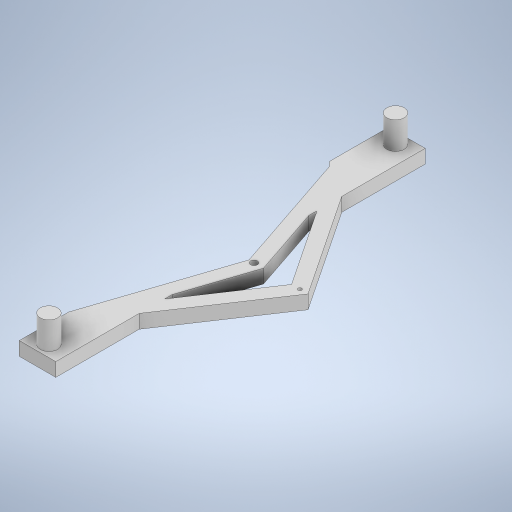
# Autodesk Inventor part: SteeringBaru
Saved by Autodesk Inventor 2024 (Build 280153000, 153)
## iProperties
Created: 2025-12-15
Part Number: SteeringBaru
Material: Generic
Document SubType Name: Modeling
Designer: risda
Density: 1 g/cm^3
Appearance: Default
Author: risda
Autodesk Inventor part; units mm, degrees
ref_plane "YZ Plane" through (0, 0, 0) normal (1, 0, 0) x (0, 1, 0)
ref_plane "XZ Plane" through (0, 0, 0) normal (0, 1, 0) x (-1, 0, 0)
ref_plane "XY Plane" through (0, 0, 0) normal (0, 0, 1) x (1, 0, 0)
sketch "Sketch1" plane through (0, 0, 0) normal (0, 1, 0) x (-1, 0, 0)
  line L0 (0, 0) -> (0, -81)
  line L1 (0, -81) -> (-8, -81)
  line L2 (-8, -81) -> (-8, 0)
  line L3 (0, 0) -> (-8, 0)
  line L4 (-4, 0) -> (-4, -2.5)
  line L5 (-4, -81) -> (-4, -78.5)
  circle A0 centre (-4, -2.5) radius 1.9
  circle A1 centre (-4, -78.5) radius 1.9
  dimension "d0" = 81
  dimension "d1" = 8
  dimension "d2" = 81
  dimension "d3" = 2.5
  dimension "d4" = 2.5
  dimension "d5" = 3.8
  dimension "d6" = 3.8
  constraints: 12 end point, 3 vertical, 2 centre point, 2 coincident, 2 midpoint, 1 horizontal, 1 perpendicular
  measures "d0" distance of L0.start L0.end
  measures "d1" distance of L0.end L1.end
  measures "d2" distance of L1.end L2.end
  measures "d3" distance of L4.start L4.end
  measures "d4" distance of L5.start L5.end
  measures "d5" diameter of A0
  measures "d6" diameter of A1
extrude "Extrusion1" add sketch "Sketch1" along normal blind 3
extrude "Extrusion2" add sketch "Sketch1" along normal blind 9 contours A0 | A1
sketch "Sketch2" plane through (0, 3, 0) normal (0, 1, 0) x (1, 0, 0)
  line L0 (8, 0) -> (8, 81) projected
  line L1 (8, 40.5) -> (18, 40.5)
  line L2 (8, 40.5) -> (8, 25.5)
  line L3 (8, 25.5) -> (0, 25.5)
  line L4 (0, 81) -> (0, 0) projected
  line L5 (8, 40.5) -> (8, 55.5)
  line L6 (8, 55.5) -> (0, 55.5)
  line L7 (0, 55.5) -> (0, 25.5)
  line L8 (8, 25.5) -> (18, 40.5)
  line L9 (8, 55.5) -> (18, 40.5)
  line L10 (8.8321, 24.9453) -> (18.8321, 39.9453)
  line L11 (8.8321, 56.0547) -> (18.8321, 41.0547)
  line L12 (8.8321, 24.9453) -> (8, 23.6972)
  line L13 (8, 23.6972) -> (8, 25.5)
  line L14 (8, 55.5) -> (8, 57.3028)
  line L15 (8.8321, 56.0547) -> (8, 57.3028)
  line L16 (18.8321, 39.9453) -> (19.2019, 40.5)
  line L17 (18.8321, 41.0547) -> (19.2019, 40.5)
  line L18 (5, 25.5) -> (5, 13.7889)
  line L19 (5, 13.7889) -> (11.3282, 23.2812)
  line L20 (11.3282, 23.2812) -> (21.3282, 38.2812)
  line L21 (21.3282, 38.2812) -> (22.8074, 40.5)
  line L22 (22.8074, 40.5) -> (21.3282, 42.7188)
  line L23 (21.3282, 42.7188) -> (11.3282, 57.7188)
  line L24 (11.3282, 57.7188) -> (5, 67.2111)
  line L25 (5, 67.2111) -> (5, 55.5)
  line L26 (8, 23.6972) -> (0, 23.6972)
  line L27 (0, 25.5) -> (0, 23.6972)
  line L28 (8, 57.3028) -> (0, 57.3028)
  line L29 (0, 57.3028) -> (0, 55.5)
  point P0 (8, 18.2889)
  point P1 (8, 62.7111)
  dimension "d11" = 10
  dimension "d12" = 15
  dimension "d13" = 15
  dimension "d14" = 1
  dimension "d15" = 1
  dimension "d16" = 3
  constraints: 56 end point, 9 point on line, 4 collinear, 4 perpendicular, 2 horizontal, 2 parallel, 1 midpoint, 1 vertical, 7 other
  measures "d11" distance of L1.start L1.end
  measures "d12" distance of L1.start L2.end
  measures "d13" distance of L1.start L5.end
  measures "d14" distance between parallel lines of L8 L10
  measures "d15" distance between parallel lines of L9 L11
  measures "d16" distance between parallel lines of L11 L23
extrude "Extrusion3" add sketch "Sketch2" against normal blind 3 contours L12 L10 L16 L17 L11 L15 L0 L24 L23 L22 L21 L20 L19
extrude "Extrusion4" cut sketch "Sketch2" against normal blind 3 contours L26 L18 L3 L0 | L3 L4 L6 L0 | L26 L4 L3 L18 | L6 L25 L28 L0 | L6 L4 L28 L25
chamfer "Chamfer1" distance 3 angle 45 2 edges at (0, 1.5, -57.3028) (0, 1.5, -23.6972)
fillet "Fillet1" radius 1 2 edges at (8, 1.5, -57.3028) (8, 1.5, -23.6972)
sketch "Sketch3" plane through (0, 3, 0) normal (0, 1, 0) x (1, 0, 0)
  line L0 (22.8074, 40.5) -> (8, 62.7111) projected
  line L1 (22.8074, 40.5) -> (21.0044, 40.5)
  circle A0 centre (21.0044, 40.5) radius 0.4
  point P0 (0, 0)
  dimension "d25" = 1.803
  dimension "d26" = 0.8
  constraints: 2 end point, 1 centre point, 1 coincident, 1 horizontal
  measures "d25" distance of L0.start L1.end
  measures "d26" diameter of A0
extrude "Extrusion5" cut sketch "Sketch3" against normal blind 3
sketch "Sketch4" plane through (0, 3, 0) normal (0, 1, 0) x (1, 0, 0)
  line L0 (0, 57.3028) -> (8.0349, 57.3028)
  line L1 (0, 57.3028) -> (0, 23.6972)
  line L2 (0, 23.6972) -> (8.0349, 23.6972)
  line L3 (8.0349, 23.6972) -> (8.0349, 57.3028)
  line L4 (0, 60.3028) -> (3, 57.3028) projected
  line L5 (0, 57.3028) -> (0, 60.3028)
  line L6 (0, 60.3028) -> (3, 57.3028)
  line L7 (0, 20.6972) -> (0, 0) projected
  line L8 (0, 20.6972) -> (0, 23.6972)
  line L9 (0, 20.6972) -> (3, 23.6972)
  line L10 (0, 57.3028) -> (8, 57.3028)
  line L11 (8, 57.3028) -> (8, 55.5125)
  line L12 (8, 55.5125) -> (0, 55.5125)
  line L13 (0, 55.5125) -> (0, 57.3028)
  line L14 (8, 55.5125) -> (13.0424, 40.5013)
  line L15 (13.0424, 40.5013) -> (8.0349, 25.4511)
  line L16 (4.5889, 24.5965) -> (9.8792, 40.4967)
  line L17 (9.8792, 40.4967) -> (4.5467, 56.3715)
  circle A0 centre (10.9842, 40.4967) radius 0.75
  line L18 (9.8792, 40.4967) -> (8.0349, 40.5)
  line L19 (9.8792, 40.4967) -> (10.9842, 40.4967)
  point P0 (8.0349, 45.9872)
  point P1 (8.0349, 34.9536)
  dimension "d29" = 8
  dimension "d30" = 3
  dimension "d31" = 1.5
  dimension "d36" = 1.8443
  dimension "d37" = 1.105
  constraints: 36 end point, 3 horizontal, 3 perpendicular, 2 collinear, 2 parallel, 2 point on line, 2 vertical, 1 centre point, 1 midpoint, 1 other
  measures "d29" distance of L11.end L12.end
  measures "d30" distance between parallel lines of L15 L16
  measures "d31" diameter of A0
  measures "d36" distance of L16.end L18.end
  measures "d37" distance of L16.end L19.end
extrude "Extrusion6" add sketch "Sketch4" against normal blind 3 contours L5 L4 L0 | L0 L11 L12 L1 | L12 L17 L3 L2 L1 | L2 L9 L8 | L12 L14 L3 L17 | L3 L14 L15 L16 L17
sketch "Sketch5" plane through (0, 3, 0) normal (0, 1, 0) x (1, 0, 0)
  line L0 (8.0349, 45.9872) -> (8.0349, 34.9536) projected
  line L1 (8.0349, 34.9536) -> (0.9671, 13.7113)
  line L2 (9.8792, 40.4967) -> (8.0349, 34.9536) projected
  line L3 (9.8792, 40.4967) -> (8.0349, 45.9872) projected
  line L4 (9.8792, 40.4967) -> (0.9671, 67.0279)
  line L5 (0.9671, 67.0279) -> (0.9671, 13.7113)
  line L6 (0, 81) -> (0, 0) projected
  line L7 (8.0349, 45.9872) -> (8.0349, 34.9536)
  point P0 (8.0349, 45.9872)
  constraints: 8 end point, 2 collinear, 2 vertical, 1 other
extrude "Extrusion7" cut sketch "Sketch5" against normal blind 3 contours L0 L1 L5 L4
sketch "Sketch6" plane through (0, 3, 0) normal (0, 1, 0) x (1, 0, 0)
  line L0 (9.8792, 40.4967) -> (0.9671, 67.0279) projected
  line L1 (0.9671, 67.0279) -> (0, 68.0001)
  line L2 (0, 81) -> (0, 0) projected
  line L3 (9.8792, 40.4967) -> (0.9671, 13.7113) projected
  line L4 (0.9671, 13.7113) -> (0, 10.8046)
  line L5 (0.9671, 13.7113) -> (0.9671, 67.0279)
  line L6 (0, 68.0001) -> (0, 10.8046)
  point P0 (0, 63.7751)
  point P1 (0, 17.0581)
  constraints: 8 end point, 2 parallel, 2 point on line, 3 other
extrude "Extrusion8" cut sketch "Sketch6" against normal blind 3 contours L5 L4 L2 L1
body "Solid1"
